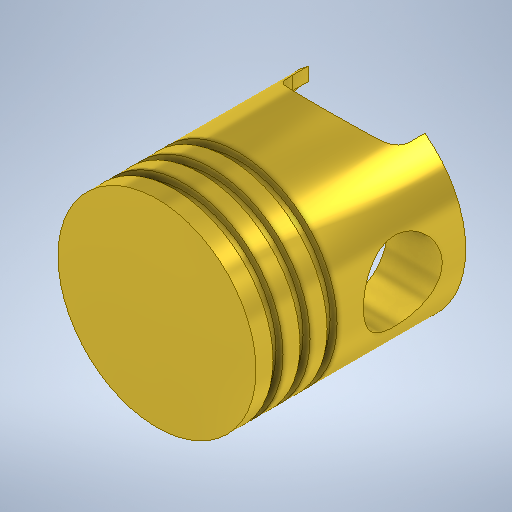
# Autodesk Inventor part: Part 1 Piston
Saved by Autodesk Inventor 2025.2 (Build 292293000, 293)
## iProperties
Created: 2025-03-19
Part Number: Part 1 Piston
Material: Stainless Steel
Document SubType Name: Sheet Metal
Designer: User
Density: 8 g/cm^3
Sheet Metal Rule: Default_mm
Appearance: Metal 2400F Hot
Author: User
Autodesk Inventor part; units mm, degrees
ref_plane "XZ Plane" through (0, 0, 0) normal (0, 1, 0) x (-1, 0, 0)
sketch "Sketch1" plane through (0, 0, 0) normal (0, 0, 1) x (1, 0, 0)
  circle A0 centre (0, 0) radius 42.5
  dimension "d0" = 85
  constraints: 1 centre point, 1 coincident
  measures "d0" diameter of A0
extrude "Extrusion1" add sketch "Sketch1" along normal blind 90
sketch "Sketch2" plane through (0, 0, 90) normal (0, 0, 1) x (1, 0, 0)
  point P0 (0, 0)
ref_plane "Work Plane1" through (0, 0, 82.7) normal (0, 0, 1) x (1, 0, 0)
sketch "Sketch3" plane through (0, 0, 82.7) normal (0, 0, 1) x (1, 0, 0)
  circle A0 centre (0, 0) radius 42.5 projected
  circle A1 centre (0, 0) radius 39.5
  dimension "d4" = 79
  constraints: 1 centre point, 1 coincident
  measures "d4" diameter of A1
extrude "Extrusion2" cut sketch "Sketch3" against normal blind 4.3
pattern_linear "Rectangular Pattern1" count 3 spacing 11.6 along (0, 0, -1) of "Extrusion2"
sketch "Sketch4" plane through (0, 0, 0) normal (0, 0, -1) x (-1, 0, 0)
  circle A0 centre (0, 0) radius 38
  dimension "d10" = 76
  constraints: 1 centre point, 1 coincident
  measures "d10" diameter of A0
extrude "Extrusion3" cut sketch "Sketch4" against normal blind 85
sketch "Sketch5" plane through (0, 0, 0) normal (1, 0, 0) x (0, 1, 0)
  circle A0 centre (0, 27) radius 16.9
  line L0 (42.5, 0) -> (-42.5, 0) projected
  point P0 (0, 0)
  dimension "d13" = 33.8
  dimension "d14" = 27
  constraints: 1 centre point
  measures "d13" diameter of A0
  measures "d14" distance from line of L0 A0.centre
extrude "Extrusion4" cut sketch "Sketch5" along normal mid plane 85
sketch "Sketch6" plane through (0, 0, 0) normal (0, 1, 0) x (-1, 0, 0)
  line L0 (38, 0) -> (-38, 0) projected
  line L1 (25, 12) -> (25, 0)
  line L2 (25, 0) -> (-25, 0)
  line L3 (-25, 0) -> (-25, 12)
  line L4 (42.5, 0) -> (-42.5, 0) projected
  arc A0 (25, 12) -> (-25, 12) centre (0, -19.225) ccw
  point P0 (0, 0)
  point P1 (0, 12)
  point P2 (0, 0)
  point P3 (-25, 0)
  dimension "d17" = 50
  dimension "d18" = 12
  dimension "d19" = 40
  constraints: 6 end point, 2 point on circle, 1 centre point, 1 midpoint, 1 parallel, 1 point on line, 1 vertical alignment
  measures "d17" distance of L1.end L2.end
  measures "d18" distance of L1.end L1.start
  measures "d19" radius of A0
extrude "Extrusion5" cut sketch "Sketch6" along normal mid plane 85
ref_plane "Work Plane2" through (-19, 0, 0) normal (1, 0, 0) x (0, 1, 0)
sketch "Sketch7" plane through (-19, 0, 0) normal (1, 0, 0) x (0, 1, 0)
  spline S0 degree 5 poles (16.9, 27) (16.8998, 30.2633) (16.113, 33.526) (14.5358, 36.536) (9.4975, 42.1791) (2.1833, 44.5372) (-2.1811, 44.5373) (-9.4958, 42.1803) (-14.5349, 36.5374) (-16.1124, 33.5277) (-17.6871, 27.0012) (-16.1132, 20.4744) (-14.5362, 17.4646) (-9.4977, 11.8209) (-2.1833, 9.4629) (2.1814, 9.4625) (9.4963, 11.8201) (14.5353, 17.4631) (16.1129, 20.4734) (16.8998, 23.7364) (16.9, 27) knots 0 0 0 0 0 0 0.153654 0.153654 0.153654 0.346327 0.346327 0.346327 0.49999 0.49999 0.49999 0.653651 0.653651 0.653651 0.846332 0.846332 0.846332 1 1 1 1 1 1 projected
  circle A0 centre (0, 27) radius 22.5
  point P0 (0, 0)
  dimension "d23" = 45
  constraints: 1 centre point, 1 other
  measures "d23" diameter of A0
extrude "Extrusion6" add sketch "Sketch7" against normal up to next
mirror "Mirror1" about plane through (0, 0, 0) normal (1, 0, 0) of "Extrusion6"
fillet "Fillet1" radius 3 4 edges at (-30.6227, -22.5, 26.9924) (-33.9337, 17.1028, 41.62) (-33.9337, 17.1027, 12.3799) (30.6227, -22.5, 26.985)
fillet "Fillet2" radius 10 4 edges at (-25, -31.4937, 12) (-25, 31.4937, 12) (25, 31.4937, 12) (25, -31.4937, 12)
sketch "Sketch8" plane through (0, 0, 0) normal (0, 1, 0) x (-1, 0, 0)
  line L0 (0, 90) -> (0, 95)
  line L1 (42.5, 90) -> (-42.5, 90) projected
  arc A0 (42.5, 90) -> (0, 95) centre (0, -88.125) ccw
  line L2 (0, 95) -> (27.9027, 95) construction
  point P0 (0, 0)
  dimension "d28" = 5
  constraints: 4 end point, 2 midpoint, 2 point on circle, 1 centre point, 1 horizontal, 1 tangent, 1 vertical
  measures "d28" distance of point (0, 90) L0.end
revolve "Revolution1" add sketch "Sketch8" angle 360 about axis through (0, 0, 90) along (0, 0, 1)
ref_plane "Work Plane3" through (0, 0, 0) normal (1, 0, 0) x (0, 1, 0)
equation "\"BendRadius\" = Thickness"
equation "\"BendReliefWidth\" = Thickness"
equation "\"BendReliefDepth\" = 0.5 * Thickness"
equation "\"CornerReliefSize\" = 4 * Thickness"
equation "\"MinimumRemnant\" = 2 * Thickness"
equation "\"TransitionRadius\" = BendRadius"
equation "\"JacobiRadiusSize\" = BendRadius"
equation "\"GapSize\" = Thickness"
equation "\"Thickness\" = 0.5"
body "Solid1"
